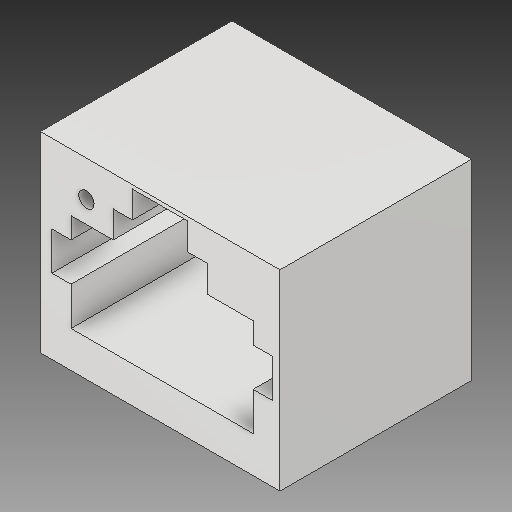
# Autodesk Inventor part: Ethernet Port
Saved by Autodesk Inventor 2017 (Build 210142000, 142)
## iProperties
Created: 2020-02-22
Part Number: Ethernet Port
Material: Acetal Resin, White
Document SubType Name: Modeling
Designer: S332848902
Density: 1.425 g/cm^3
Appearance: Smooth - White
Author: S332848902
Autodesk Inventor part; units mm, degrees
ref_plane "YZ Plane" through (0, 0, 0) normal (1, 0, 0) x (0, 1, 0)
ref_plane "XZ Plane" through (0, 0, 0) normal (0, 1, 0) x (-1, 0, 0)
ref_plane "XY Plane" through (0, 0, 0) normal (0, 0, 1) x (1, 0, 0)
sketch "Sketch1" plane through (0, 0, 0) normal (0, 0, 1) x (1, 0, 0)
  point P0 (0, 0)
sketch "Sketch2" plane through (0, 0, 0) normal (0, 0, 1) x (1, 0, 0)
  line L0 (0, 0) -> (15.875, 0)
  line L1 (15.875, 0) -> (15.875, 12.7)
  line L2 (15.875, 12.7) -> (0, 12.7)
  line L3 (0, 12.7) -> (0, 0)
  dimension "d0" = 15.875
  dimension "d1" = 12.7
  constraints: 8 end point, 2 parallel, 1 horizontal, 1 perpendicular
  measures "d0" distance of L2.end L1.end
  measures "d1" distance of L1.end L0.end
extrude "Extrusion1" add sketch "Sketch2" along normal blind 12.7
sketch "Sketch3" plane through (0, 0, 12.7) normal (0, 0, 1) x (1, 0, 0)
  line L0 (0, 12.7) -> (0, 0) projected
  line L1 (0, 0) -> (2.032, 0)
  line L2 (0, 0) -> (15.875, 0) projected
  line L3 (2.032, 2.413) -> (14.097, 2.413)
  line L4 (14.097, 2.413) -> (14.097, 8.89)
  line L5 (14.097, 8.89) -> (2.032, 8.89)
  line L6 (2.032, 8.89) -> (2.032, 2.413)
  constraints: 10 end point, 2 perpendicular, 1 parallel, 1 point on line
extrude "Extrusion2" cut sketch "Sketch3" against normal blind 10.16
sketch "Sketch4" plane through (0, 0, 12.7) normal (0, 0, 1) x (1, 0, 0)
  line L0 (2.032, 8.89) -> (14.097, 8.89) projected
  line L1 (11.049, 8.89) -> (11.049, 10.668)
  line L2 (11.049, 10.668) -> (4.826, 10.668)
  line L3 (4.826, 10.668) -> (4.826, 8.89)
  line L4 (11.049, 8.89) -> (4.826, 8.89)
  point P0 (0, 0)
  dimension "d13" = 3.048
  dimension "d16" = 6.223
  constraints: 8 end point, 3 perpendicular, 2 point on line
  measures "d13" distance of L0.end L1.start
  measures "d16" distance of L1.end L2.end
extrude "Extrusion3" cut sketch "Sketch4" against normal blind 10.16
sketch "Sketch5" plane through (0, 0, 12.7) normal (0, 0, 1) x (1, 0, 0)
  line L0 (11.049, 10.668) -> (11.049, 8.89) projected
  line L1 (4.826, 10.668) -> (11.049, 10.668) projected
  line L2 (9.779, 10.668) -> (9.779, 12.446)
  line L3 (9.779, 12.446) -> (6.096, 12.446)
  line L4 (6.096, 12.446) -> (6.096, 10.668)
  line L5 (6.096, 10.668) -> (9.779, 10.668)
  point P0 (0, 0)
  constraints: 8 end point, 2 perpendicular, 2 point on line, 1 collinear
extrude "Extrusion4" cut sketch "Sketch5" against normal blind 10.16
sketch "Sketch6" plane through (0, 0, 12.7) normal (0, 0, 1) x (1, 0, 0)
  line L0 (14.097, 2.413) -> (2.032, 2.413) projected
  line L1 (14.097, 8.89) -> (14.097, 2.413) projected
  line L2 (14.097, 4.953) -> (15.367, 4.953)
  line L3 (15.367, 4.953) -> (15.367, 7.493)
  line L4 (15.367, 7.493) -> (14.097, 7.493)
  line L5 (14.097, 7.493) -> (14.097, 4.953)
  line L6 (2.032, 2.413) -> (2.032, 8.89) projected
  line L7 (2.032, 4.953) -> (0.762, 4.953)
  line L8 (0.762, 4.953) -> (0.762, 7.493)
  line L9 (0.762, 7.493) -> (2.032, 7.493)
  line L10 (2.032, 7.493) -> (2.032, 4.953)
  point P0 (0, 0)
  constraints: 16 end point, 4 perpendicular, 4 point on line, 2 horizontal, 1 collinear
extrude "Extrusion5" cut sketch "Sketch6" against normal blind 10.16
sketch "Sketch7" plane through (0, 0, 12.7) normal (0, 0, 1) x (1, 0, 0)
  circle A0 centre (3.0514, 10.3254) radius 0.508
  point P0 (0, 0)
  dimension "d33" = 1.016
  constraints: 1 centre point
  measures "d33" diameter of A0
extrude "Extrusion6" cut sketch "Sketch7" against normal blind 10.16
body "Solid1"
